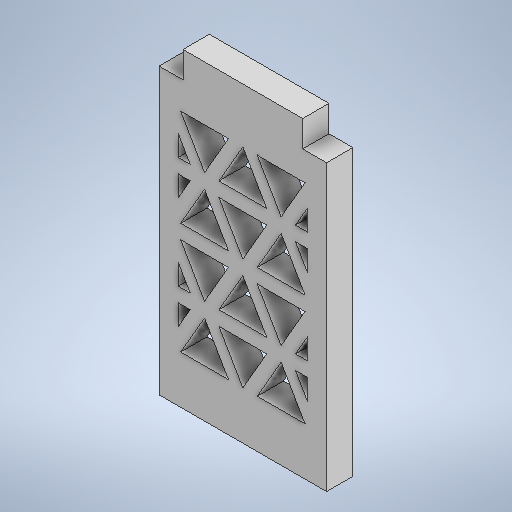
# Autodesk Inventor part: motor_setter_spacer
Saved by Autodesk Inventor 2026.1 (Build 301233020, 233B)
## iProperties
Created: 2025-10-31
Part Number: motor_setter_spacer
Material: 一般
Document SubType Name: Modeling
Designer: hibik
Density: 1 g/cm^3
Appearance: 既定
Author: hibik
Autodesk Inventor part; units mm, degrees
ref_plane "YZ Plane" through (0, 0, 0) normal (1, 0, 0) x (0, 1, 0)
ref_plane "XZ Plane" through (0, 0, 0) normal (0, 1, 0) x (-1, 0, 0)
sketch "スケッチ1" plane through (0, 0, 0) normal (0, 0, 1) x (1, 0, 0)
  line L0 (-17.5, 0) -> (17.5, 0)
  line L1 (17.5, 0) -> (17.5, 59.5)
  line L2 (17.5, 59.5) -> (-17.5, 59.5)
  line L3 (-17.5, 59.5) -> (-17.5, 0)
  line L4 (-12.5, 59.5) -> (12.5, 59.5)
  line L5 (12.5, 59.5) -> (12.5, 65)
  line L6 (12.5, 65) -> (-12.5, 65)
  line L7 (-12.5, 65) -> (-12.5, 59.5)
  point P0 (0, 0)
  point P1 (0, 0)
  point P2 (0, 59.5)
  dimension "d0" = 59.5
  dimension "d1" = 35
  dimension "d2" = 25
  dimension "d3" = 5.5
  constraints: 16 end point, 4 parallel, 3 midpoint, 2 horizontal, 2 perpendicular, 1 coincident, 1 point on line
  measures "d0" distance of L2.end L0.start
  measures "d1" distance of L1.end L2.end
  measures "d2" distance of L5.end L6.end
  measures "d3" distance of L4.end L5.end
extrude "押し出し1" add sketch "スケッチ1" along normal blind 5.5
sketch "スケッチ2" plane through (0, 0, 5.5) normal (0, 0, 1) x (1, 0, 0)
  line L0 (-13, 10) -> (-3, 10)
  line L1 (-13, 10) -> (-8, 18.6603)
  line L2 (-8, 18.6603) -> (-3, 10)
  line L3 (0, 10) -> (5, 18.6603)
  line L4 (5, 18.6603) -> (-5, 18.6603)
  line L5 (-5, 18.6603) -> (0, 10)
  line L6 (3, 10) -> (13, 10)
  line L7 (13, 10) -> (8, 18.6603)
  line L8 (8, 18.6603) -> (3, 10)
  line L9 (0, -13) -> (0, 78) projected
  line L10 (-17.5, 0) -> (17.5, 0) projected
  line L11 (-11, 18.6603) -> (-16, 10)
  line L12 (-16, 10) -> (-16, 18.6603)
  line L13 (-16, 18.6603) -> (-11, 18.6603)
  line L14 (-13.5, 18.6603) -> (-13.5, 10)
  point P0 (0, 0)
  point P1 (0, 18.6603)
  point P2 (-13.5, 14.3301)
  dimension "d6" = 10
  dimension "d7" = 3
  dimension "d8" = 10
  dimension "d9" = 3
  constraints: 26 end point, 7 equal length, 5 point on line, 3 horizontal, 2 parallel, 2 vertical, 1 midpoint, 1 perpendicular, 1 other
  measures "d6" distance of L0.start L0.end
  measures "d7" distance from line of L9 L0.end
  measures "d8" distance between parallel lines of L10 L0
  measures "d9" distance of L1.end L11.start
extrude "押し出し2" cut sketch "スケッチ2" against normal through all contours L1 L2 L0 | L5 L4 L9 | L11 L14 L13
ref_plane "作業平面1" through (-5, 20.1603, 5.5) normal (0, -1, 0) x (1, 0, 0)
mirror "ミラー1" about plane through (-5, 20.1603, 5.5) normal (0, -1, 0) of "押し出し2"
pattern_linear "矩形状パターン1" count 2 spacing 23.3 along (0, 1, 0) of "押し出し2", "ミラー1"
mirror "ミラー2" about plane through (0, 0, 0) normal (1, 0, 0) of "押し出し2", "ミラー1", "矩形状パターン1"
equation "\"d9\" = d7"
